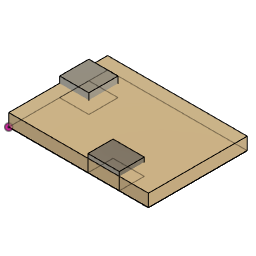
_ DCDC step down converter v1 (Autodesk Fusion 360 design; units mm, degrees)
Autodesk Fusion 360 part; units mm, degrees
sketch "Sketch1" plane through (0, 0, 0) normal (0, 0, 1) x (1, 0, 0)
  line L0 (0, 0) -> (33.5, 0)
  line L1 (33.5, 0) -> (33.5, 23.7)
  line L2 (33.5, 23.7) -> (0, 23.7)
  line L3 (0, 23.7) -> (0, 0)
  line L4 (0, 19.2) -> (7, 19.2)
  line L5 (7, 19.2) -> (7, 12.2)
  line L6 (7, 12.2) -> (0, 12.2)
  line L7 (0, 12.2) -> (0, 19.2)
  line L8 (19, 0) -> (26.5, 0)
  line L9 (26.5, 0) -> (26.5, 6)
  line L10 (26.5, 6) -> (19, 6)
  line L11 (19, 6) -> (19, 0)
  dimension "d1" = 33.5
  dimension "d2" = 23.7
  dimension "d5" = 7
  dimension "d6" = 7
  dimension "d7" = 4.5
  dimension "d8" = 7.5
  dimension "d9" = 6
  dimension "d10" = 7
  constraint horizontal L0
  constraint vertical L1
  constraint horizontal L2
  constraint vertical L3
  constraint coincident L0.start L3.end
  constraint horizontal L4
  constraint vertical L5
  constraint horizontal L6
  constraint vertical L7
  constraint coincident L3 L4.start
  constraint horizontal L8
  constraint vertical L9
  constraint horizontal L10
  constraint vertical L11
  constraint coincident L0 L8.start
  measures "d1" distance of L0.start L0.end
  measures "d2" distance of L0.start L2.end
  measures "d5" distance of L4.start L4.end
  measures "d6" distance of L4.start L6.end
  measures "d7" distance of L2 L4
  measures "d8" distance of L8.start L8.end
  measures "d9" distance of L8.start L10.end
  measures "d10" distance of L1 L9
extrude "Extrude1" add sketch "Sketch1" along normal blind 3 makes body 1
extrude "Extrude2" add sketch "Sketch1" along normal blind 4.5 separate body contours L3 L4 L5 L6 L7 makes body 2
extrude "Extrude3" add sketch "Sketch1" along normal blind 4 separate body contours L0 L8 L9 L10 L11 makes body 3
